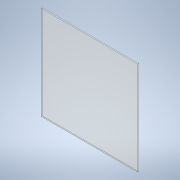
# Autodesk Inventor part: door glass
Saved by Autodesk Inventor 2020 (Build 240168000, 168)
## iProperties
Created: 2020-05-19
Part Number: door glass
Material: Glass
Document SubType Name: Modeling
Designer: kolbe
Density: 2.18 g/cm^3
Appearance: Clear
Author: kolbe
Autodesk Inventor part; units mm, degrees
ref_plane "YZ Plane" through (0, 0, 0) normal (1, 0, 0) x (0, 1, 0)
ref_plane "XZ Plane" through (0, 0, 0) normal (0, 1, 0) x (-1, 0, 0)
ref_plane "XY Plane" through (0, 0, 0) normal (0, 0, 1) x (1, 0, 0)
sketch "Sketch2" plane through (0, 0, 0) normal (0, 0, 1) x (1, 0, 0)
  line L0 (0, 0) -> (825.5, 0)
  line L1 (825.5, 0) -> (825.5, 800.1)
  line L2 (825.5, 800.1) -> (0, 800.1)
  line L3 (0, 800.1) -> (0, 0)
  dimension "d0" = 825.5
  dimension "d1" = 800.1
  constraints: 8 end point, 2 parallel, 1 horizontal, 1 perpendicular
  measures "d0" distance of L2.end L1.end
  measures "d1" distance of L1.end L0.end
extrude "Extrusion1" add sketch "Sketch2" along normal blind 9.525
body "Solid1"
